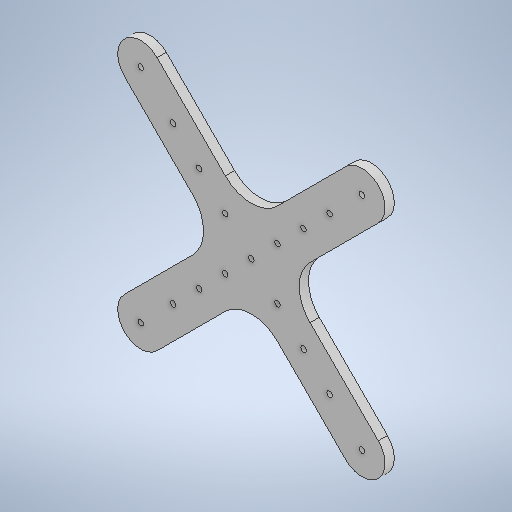
# Autodesk Inventor part: Base
Saved by Autodesk Inventor 2025.1 (Build 291241020, 241B)
## iProperties
Created: 2024-09-22
Part Number: Base
Material: 일반
Document SubType Name: Modeling
Designer: daare
Density: 1 g/cm^3
Appearance: 기본값
Author: daare
Autodesk Inventor part; units mm, degrees
ref_plane "YZ Plane" through (0, 0, 0) normal (1, 0, 0) x (0, 1, 0)
ref_plane "XZ Plane" through (0, 0, 0) normal (0, 1, 0) x (-1, 0, 0)
ref_plane "XY Plane" through (0, 0, 0) normal (0, 0, 1) x (1, 0, 0)
sketch "스케치1" plane through (0, 0, 0) normal (0, 0, 1) x (1, 0, 0)
  arc A0 (-51.1612, 68.8388) -> (-68.8388, 51.1612) centre (-60, 60) ccw
  line L0 (-68.8388, 51.1612) -> (-31.8198, 14.1421)
  line L1 (-51.1612, 68.8388) -> (-14.1421, 31.8198)
  line L2 (-60, 60) -> (0, 0)
  arc A1 (-25.9619, 0) -> (-31.8198, 14.1421) centre (-45.9619, 0) ccw
  line L3 (-93.2132, 0) -> (15.5355, 0) projected
  arc A2 (-14.1421, 31.8198) -> (0, 25.9619) centre (0, 45.9619) ccw
  line L4 (0, -15.5355) -> (0, 93.2132) projected
  dimension "d0" = 60
  dimension "d1" = 60
  dimension "d2" = 25
  dimension "d3" = 20
  constraints: 6 end point, 6 point on circle, 3 centre point, 3 symmetric about line, 3 tangent, 2 parallel, 1 horizontal alignment, 1 point on line, 1 other
  measures "d0" horizontal distance of L2.end L2.start
  measures "d1" horizontal distance of L2.end L2.start
  measures "d2" diameter of A0
  measures "d3" radius of A1
extrude "돌출1" add sketch "스케치1" along normal blind 5
pattern_circular "원형 패턴1" count 4 over 360 about axis through (0, 0, -10) along (0, 0, 1) of "돌출1"
sketch "스케치2" plane through (0, 0, 5) normal (0, 0, 1) x (1, 0, 0)
  arc A0 (-51.1612, 68.8388) -> (-68.8388, 51.1612) centre (-60, 60) ccw projected
  line L0 (-60, 60) -> (0, 0)
  point P0 (-14.1421, 14.1421)
  point P1 (-28.2843, 28.2843)
  point P2 (-42.4264, 42.4264)
  dimension "d9" = 84.8528
  dimension "d10" = 20
  dimension "d13" = 20
  constraints: 2 coincident, 2 end point, 1 point on line, 3 other
  measures "d9" distance of L0.start L0.end
  measures "d10" distance of point (0, 0) point (-14.142, 14.142)
  measures "d13" distance of point (-14.142, 14.142) point (-28.284, 28.284)
hole "구멍1" at (0, 0, 5) at (-60, 60, 5) at (-14.1421, 14.1421, 5) at (-28.2843, 28.2843, 5) at (-42.4264, 42.4264, 5) direction (0, 0, -1) diameter 3 end through all
pattern_circular "원형 패턴2" count 4 over 360 about axis through (0, 0, -10) along (0, 0, 1) of "구멍1"
equation "\"d13\" = d10"
